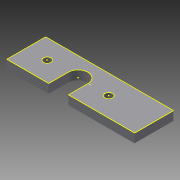
# Autodesk Inventor part: Servo Groove Mountv6
Saved by Autodesk Inventor 2013 (Build 170138000, 138)
## iProperties
Created: 2013-11-15
Part Number: Servo Groove Mountv6
Material: Generic
Document SubType Name: Modeling
Designer: Enlightx
Density: 1 g/cm^3
Author: Enlightx
Autodesk Inventor part; units mm, degrees
ref_plane "YZ Plane" through (0, 0, 0) normal (1, 0, 0) x (0, 1, 0)
ref_plane "XZ Plane" through (0, 0, 0) normal (0, 1, 0) x (-1, 0, 0)
ref_plane "XY Plane" through (0, 0, 0) normal (0, 0, 1) x (1, 0, 0)
sketch "Sketch1" plane through (0, 0, 0) normal (0, 0, 1) x (1, 0, 0)
  line L0 (-39.5, 12) -> (39.5, 12)
  line L1 (39.5, 12) -> (39.5, -12)
  line L2 (39.5, -12) -> (-39.5, -12)
  line L3 (-39.5, -12) -> (-39.5, 12)
  line L4 (-39.5, 12) -> (39.5, -12) construction
  line L5 (39.5, 12) -> (-39.5, -12) construction
  point P0 (0, 0)
  dimension "d0" = 79
  dimension "d1" = 24
  constraints: 12 end point, 2 midpoint, 2 parallel, 1 horizontal, 1 perpendicular
  measures "d0" distance of L1.end L2.end
  measures "d1" distance of L0.end L1.end
extrude "Extrusion1" add sketch "Sketch1" along normal blind 5.6
sketch "Sketch5" plane through (0, 0, 0) normal (0, 0, -1) x (-1, 0, 0)
  line L0 (-39.5, -12) -> (39.5, -12) projected
  line L1 (39.5, 12) -> (-24.5, 12) construction
  line L2 (-24.5, 12) -> (-24.5, -12) construction
  line L3 (-24.5, -12) -> (39.5, -12) construction
  line L4 (39.5, -12) -> (39.5, 12) construction
  line L5 (-24.5, 12) -> (39.5, -12) construction
  line L6 (39.5, 12) -> (-24.5, -12) construction
  circle A0 centre (7.5, 0) radius 6.1
  line L7 (-11.5, 3) -> (26.5, 3) construction
  line L8 (26.5, 3) -> (26.5, -3) construction
  line L9 (26.5, -3) -> (-11.5, -3) construction
  line L10 (-11.5, -3) -> (-11.5, 3) construction
  line L11 (-11.5, 3) -> (26.5, -3) construction
  line L12 (26.5, 3) -> (-11.5, -3) construction
  circle A1 centre (-11.5, 0) radius 2.4
  circle A2 centre (26.5, 0) radius 2.4
  line L13 (1.4, 0) -> (1.4, -12)
  line L14 (13.6, 0) -> (13.6, -12)
  line L15 (13.6, -12) -> (1.4, -12)
  line L16 (-15, 12) -> (30, 12) construction
  line L17 (30, 12) -> (30, -12) construction
  line L18 (30, -12) -> (-15, -12) construction
  line L19 (-15, -12) -> (-15, 12) construction
  line L20 (-15, 12) -> (30, -12) construction
  line L21 (30, 12) -> (-15, -12) construction
  point P0 (-25, -12)
  point P1 (0, 0)
  dimension "d29" = 64
  dimension "d30" = 12.2
  dimension "d31" = 38
  dimension "d32" = 4.8
  dimension "d33" = 4.8
  constraints: 42 end point, 7 midpoint, 6 parallel, 5 perpendicular, 4 point on line, 3 centre point, 3 horizontal, 2 point on circle, 2 tangent, 1 collinear
  measures "d29" distance of L3.end L2.end
  measures "d30" diameter of A0
  measures "d31" distance of L8.end L9.end
  measures "d32" diameter of A1
  measures "d33" diameter of A2
extrude "Extrusion4" cut sketch "Sketch5" against normal blind 5.6
sketch "Sketch7" plane through (0, 0, 5.6) normal (0, 0, 1) x (1, 0, 0)
  line L0 (-1.4, 0) -> (-1.4, -12) projected
  line L1 (-1.4, -12) -> (39.5, -12) projected
  line L2 (39.5, -12) -> (39.5, 12) projected
  line L3 (39.5, 12) -> (-39.5, 12) projected
  line L4 (-39.5, 12) -> (-39.5, -12) projected
  line L5 (-39.5, -12) -> (-13.6, -12) projected
  line L6 (-13.6, -12) -> (-13.6, 0) projected
  arc A0 (-1.4, 0) -> (-13.6, 0) centre (-7.5, 0) ccw projected
  circle A1 centre (11.5, 0) radius 2.4 projected
  circle A2 centre (-26.5, 0) radius 2.4 projected
  point P0 (0, 0)
body "Solid1"
